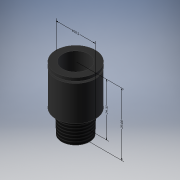
# Autodesk Inventor part: KQ2S12-02AS (A) Brass
Saved by Autodesk Inventor 2024.3 (Build 283343000, 343)
## iProperties
Created: 2024-01-12
Part Number: KQ2S12-02AS (A) Brass
Material: Generic
Catalog Web Link: www.cadenas.de
Description: KQ2S-Hex. Socket Head Male Connector (Sealant)
Vendor: SMC
Document SubType Name: Modeling
Designer: psAdmin
Manufacturer: SMC
Mass: 21 g
Surface Area: 30.0748 cm^2
Volume: 3.96052 cm^3
Density: 1 g/cm^3
Appearance: PSOLRGB-175-175-175
Category: PARTsolutions
Company: SMC
PSOL_IDENT_0: {$CADENAS_DATA/23d-libs/smc_jp/fittings_and_tubing/fittings_for_general_purposes/kq2_new/kq2_1/kq2s_
PSOL_IDENT_1: hshmc_s.prj},174 {VTYP=3D},{NB=KQ2S12-02AS},{LINA=KQ2S12-02AS},{NN=KQ2S},{DATE=07.12.2023 03:14:12},
PSOL_IDENT_2: {GEOMDATE=11.09.2019 04:59:54},{VERSION=},{LINEID=210},{WBVAR=MATERIAL,SEAL},{WBNUMERIC=}  {NB=KQ2S1
PSOL_IDENT_3: 2-02AS},{LINA=KQ2S12-02AS},{KT=DUMMY},{GUI=KQ2S12-02},{OD=12},{T=1/4},{RA=13.157},{RD=9.4},{RL=10.5}
PSOL_IDENT_4: ,{MODEL=KQ2S12-02AS},{MATERIAL=A},{MATERIALX='A','(A) Brass','N','(N) Brass + With electroless nicke
PSOL_IDENT_5: l plating'},{SEAL=S},{TUBE=12},{PORT=02},{H=8},{D=18.2},{L1=29.0},{L2=21.5},{A=24.3},{M=17.0},{EA1=4
PSOL_IDENT_6: 6.0},{EA2=44.5},{MBS=8.1},{CNSMASSEXACT=21.0},{NENN=KQ2S12-02AS},{A1=18.2},{A2=12.95},{TA=6.010},{OR
PSOL_IDENT_7: DER=KQ2S12-02AS}
NB: KQ2S12-02AS
NN: KQ2S
NT: Hex. Socket Head Male Connector (Sealant)
NBSYN: $MODEL.
LINA: KQ2S12-02AS
CATALOG: SMC (JP
ROWDESC: KQ2S12-02AS
GUI: KQ2S12-02
OD: 12
T: 1/4
MODEL: KQ2S12-02AS
MATERIAL: (A) Brass
SEAL: (S) With seal
H: 8
D: 18.2
L1: 29
L2: 21.5
A: 24.3
M: 17
EA1: 46
EA2: 44.5
MBS: 8.1
CNSMASSEXACT: 21
SUPPLIER: SMC
ARTICLENO: KQ2S12-02AS
BOMINFO: KQ2S12-02AS
CREATOR: CADENAS GmbH
Title: KQ2S12-02AS
Author: Cadenas PARTsolutions
Comments: Hex. Socket Head Male Connector (Sealant)
Autodesk Inventor part; units mm, degrees
sketch "Sketch_1" plane through (0, 0, 0) normal (0, 0, 1) x (1, 0, 0)
  line L0 (0, -6.01) -> (0, 24.3)
  line L1 (0, 24.3) -> (9.1, 24.3)
  line L2 (9.1, 24.3) -> (9.1, 22.8)
  line L3 (9.1, 22.8) -> (6.475, 22.8)
  line L4 (6.475, 22.8) -> (6.475, 21.9)
  line L5 (6.475, 21.9) -> (9.1, 21.9)
  line L6 (9.1, 21.9) -> (9.1, 5.8)
  line L7 (9.1, 5.8) -> (6.7596, 5.8)
  line L8 (6.7596, 5.8) -> (6.3909, -6.01)
  line L9 (6.3909, -6.01) -> (0, -6.01)
  line L10 (0, -6.01) -> (0, 24.3)
  constraints: 22 end point
revolve "Revolution1" add sketch "Sketch_1" angle 360 about axis through (0, -6.01, 0) along (0, -1, 0)
thread "Thread1" size "R 1/4" standard "ISO Taper" full length
sketch "_____1" plane through (0, 0, 0) normal (0, 0, 1) x (1, 0, 0)
  line L0 (-13.157, -4.7) -> (-13.157, -6.01)
  line L1 (-13.157, -6.01) -> (13.157, -6.01)
  line L2 (13.157, -6.01) -> (13.157, -4.7)
  line L3 (13.157, -4.7) -> (-13.157, -4.7)
  constraints: 8 end point
extrude "Extrusion1" cut sketch "_____1" along normal mid plane 26.314
sketch "Sketch_2" plane through (0, 0, 0) normal (0, 0, 1) x (1, 0, 0)
  line L0 (0, 7.3) -> (0, 24.3)
  line L1 (0, 24.3) -> (6, 24.3)
  line L2 (6, 24.3) -> (6, 7.3)
  line L3 (6, 7.3) -> (0, 7.3)
  line L4 (0, 7.3) -> (0, 24.3)
  constraints: 10 end point
revolve "Revolution2" cut sketch "Sketch_2" angle 360 about axis through (0, 7.3, 0) along (0, -1, 0)
sketch "Sketch_3" plane through (0, 24.3, 0) normal (0, 1, 0) x (1, 0, 0)
  line L0 (-4, -2.3094) -> (0, -4.6188)
  line L1 (0, -4.6188) -> (4, -2.3094)
  line L2 (4, -2.3094) -> (4, 2.3094)
  line L3 (4, 2.3094) -> (0, 4.6188)
  line L4 (0, 4.6188) -> (-4, 2.3094)
  line L5 (-4, 2.3094) -> (-4, -2.3094)
  constraints: 12 end point
extrude "Extrusion2" cut sketch "Sketch_3" against normal blind 21.5
ref_plane "CNS_SCREW_XY" through (0, 0, 0) normal (0, 1, 0) x (1, 0, 0)
ref_plane "CNS_SCREW_YZ" through (0, 0, 0) normal (1, 0, 0) x (0, 0, -1)
ref_plane "CNS_SCREW_ZX" through (0, 0, 0) normal (0, 0, -1) x (0, 1, 0)
body "Solid1"
